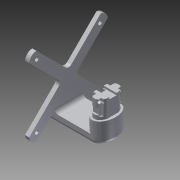
# Autodesk Inventor part: monitor-mount
Saved by Autodesk Inventor 2015 (Build 190159000, 159)
## iProperties
Created: 2015-03-06
Part Number: monitor-mount
Material: ABS Plastic
Document SubType Name: Modeling
Designer: Jody
Density: 1.06 g/cm^3
Appearance: Smooth - White
Mass: 59.874 g
Surface Area: 171.606 cm^2
Volume: 56.4849 cm^3
Author: Jody
Autodesk Inventor part; units mm, degrees
ref_plane "YZ Plane" through (0, 0, 0) normal (1, 0, 0) x (0, 1, 0)
ref_plane "XZ Plane" through (0, 0, 0) normal (0, 1, 0) x (-1, 0, 0)
ref_plane "XY Plane" through (0, 0, 0) normal (0, 0, 1) x (1, 0, 0)
sketch "Sketch1" plane through (0, 0, 0) normal (0, 1, 0) x (-1, 0, 0)
  ellipse E0 centre (0, 0) end of major axis (0, -16.9) minor radius 10.95
  dimension "d0" = 16.9
  dimension "d1" = 10.95
  constraints: 1 coincident, 2 other
extrude "Extrusion1" add sketch "Sketch1" along normal blind 25
sketch "Sketch2" plane through (0, 25, 0) normal (0, 1, 0) x (1, 0, 0)
  line L0 (7.6, 6.869) -> (7.6, -6.8693)
  line L1 (-7.6, -6.8693) -> (-7.6, 6.869)
  line L2 (1.547, -14.35) -> (-1.547, -14.35)
  line L3 (-1.547, 14.35) -> (1.547, 14.35)
  spline S0 degree 5 poles (7.6, 6.869) (7.3339, 7.69) (6.6747, 9.389) (5.6155, 11.3113) (4.2798, 12.863) (2.8086, 13.8602) (1.8557, 14.2496) (1.547, 14.35) knots 0 0 0 0 0 0 0.371815 0.797909 1 1 1 1 1 1
  line L4 (7.9552, 5.7734) -> (7.2448, 7.9647) construction
  arc A0 (7.863, 5.9868) -> (7.2954, 7.7378) centre (-10.8296, 0.8944) ccw construction
  spline S1 degree 5 poles (-1.547, 14.35) (-1.8557, 14.2496) (-2.8086, 13.8602) (-4.2798, 12.863) (-5.6155, 11.3113) (-6.6747, 9.389) (-7.3339, 7.69) (-7.6, 6.869) knots 0 0 0 0 0 0 0.202091 0.628185 1 1 1 1 1 1
  line L5 (-7.2448, 7.9647) -> (-7.9552, 5.7734) construction
  arc A1 (-7.2954, 7.7378) -> (-7.863, 5.9868) centre (10.8296, 0.8944) ccw construction
  spline S2 degree 5 poles (-7.6, -6.8693) (-7.3341, -7.6901) (-6.733, -9.2397) (-5.6943, -11.1801) (-4.3754, -12.7614) (-2.913, -13.7987) (-1.9626, -14.2149) (-1.547, -14.35) knots 0 0 0 0 0 0 0.37178 0.727887 1 1 1 1 1 1
  spline S3 degree 5 poles (1.547, -14.35) (1.9626, -14.2149) (2.913, -13.7987) (4.3754, -12.7614) (5.6943, -11.1801) (6.733, -9.2397) (7.3341, -7.6901) (7.6, -6.8693) knots 0 0 0 0 0 0 0.272113 0.62822 1 1 1 1 1 1
  line L6 (-2.5566, -14.0218) -> (-0.5374, -14.6782) construction
  arc A2 (-2.3246, -14.0283) -> (-0.7288, -14.5471) centre (0.1247, -9.2081) ccw construction
  line L7 (0.5374, -14.6782) -> (2.5566, -14.0218) construction
  arc A3 (0.7288, -14.5471) -> (2.3246, -14.0283) centre (-0.1247, -9.2081) ccw construction
  point P0 (5.4887, -11.1759)
  point P1 (2.672, 13.8453)
  point P2 (-5.4887, 11.1759)
  point P3 (-2.672, -13.8453)
  constraints: 24 end point, 8 midpoint, 4 centre point, 4 point on circle, 2 parallel, 1 horizontal, 1 perpendicular, 24 other
extrude "Extrusion3" add sketch "Sketch2" along normal blind 21
sketch "Sketch6" plane through (0, 46, 0) normal (0, 1, 0) x (1, 0, 0)
  line L0 (3.7, -9.8) -> (10.95, -9.8)
  line L1 (-10.95, -8.35) -> (-3.7, -8.35)
  line L2 (-3.7, -8.35) -> (-3.7, -16.9)
  line L3 (3.7, -9.8) -> (3.7, -16.9)
  line L4 (-3.7, -16.9) -> (-10.95, -8.35)
  line L5 (3.7, -16.9) -> (10.95, -9.8)
  line L6 (3.7, 9.8) -> (10.95, 9.8)
  line L7 (-10.95, 8.35) -> (-3.7, 8.35)
  line L8 (-3.7, 8.35) -> (-3.7, 16.9)
  line L9 (3.7, 9.8) -> (3.7, 16.9)
  line L10 (-3.7, 16.9) -> (-10.95, 8.35)
  line L11 (3.7, 16.9) -> (10.95, 9.8)
  point P0 (0, 0)
  constraints: 24 end point
extrude "Extrusion4" cut sketch "Sketch6" against normal blind 17.7
sketch "Sketch7" plane through (0, 46, 0) normal (0, 1, 0) x (1, 0, 0)
  ellipse E0 centre (0, 0) end of major axis (0, -16.9) minor radius 10.95 projected
  line L0 (10.581, -4.35) -> (-10.581, -4.35)
  line L1 (-10.581, -4.35) -> (-10.581, 4.35)
  line L2 (-10.581, 4.35) -> (10.581, 4.35)
  line L3 (10.581, 4.35) -> (10.581, -4.35)
  line L4 (10.581, -4.35) -> (-10.581, 4.35) construction
  line L5 (-10.581, -4.35) -> (10.581, 4.35) construction
  dimension "d23" = 8.7
  constraints: 12 end point, 2 midpoint, 2 parallel, 1 horizontal, 1 perpendicular, 2 other
  measures "d23" distance of L0.end L1.end
extrude "Extrusion5" cut sketch "Sketch7" against normal blind 2.4 contours L0 L1 L2 L3
sketch "Sketch8" plane through (7.6, 25, 6.8693) normal (1, 0, 0) x (0, 0, -1)
  line L0 (-7.4807, 4.8) -> (-7.4807, 12.1)
  line L1 (-5.4807, 4.8) -> (-5.4807, 12.1)
  line L2 (-7.4807, 4.8) -> (-5.4807, 4.8)
  line L3 (-5.4807, 12.1) -> (-7.4807, 12.1)
  line L4 (21.2193, 4.8) -> (21.2193, 12.1)
  line L5 (19.2193, 4.8) -> (19.2193, 12.1)
  line L6 (21.2193, 4.8) -> (19.2193, 4.8)
  line L7 (19.2193, 12.1) -> (21.2193, 12.1)
  point P0 (6.8693, -25)
  point P1 (0, 0)
  constraints: 16 end point, 2 horizontal
extrude "Extrusion6" cut sketch "Sketch8" against normal up to next
sketch "Sketch9" plane through (-7.6, 25, -6.869) normal (-1, 0, 0) x (0, 0, 1)
  line L0 (3.4692, 5) -> (10.2692, 5)
  line L1 (3.4692, 5) -> (3.4692, 18.6)
  line L2 (10.2692, 5) -> (10.2692, 18.6)
  line L3 (3.4692, 18.6) -> (10.2692, 18.6)
  point P0 (6.869, -25)
  constraints: 8 end point, 1 perpendicular
extrude "Extrusion7" cut sketch "Sketch9" against normal blind 3.5
sketch "Sketch10" plane through (-7.6, 30, -3.3999) normal (0, 0, 1) x (1, 0, 0)
  line L0 (0, 0) -> (3.5, 7.1937)
  line L1 (3.5, 0) -> (3.5, 13.6) projected
  line L2 (3.5, 7.1937) -> (3.5, 8.6937)
  line L3 (3.5, 8.6937) -> (0.864, 10.4946)
  line L4 (0, 0) -> (3.5, 0)
  line L5 (0, 0) -> (3.5, 0) projected
  line L6 (0.864, 10.4946) -> (3.5, 13.6)
  point P0 (7.6, -30)
  dimension "d36" = 8
  dimension "d37" = 1.5
  constraints: 10 end point, 2 point on line, 1 collinear
  measures "d36" distance of L0.start L0.end
  measures "d37" distance of L0.end L2.end
extrude "Extrusion8" add sketch "Sketch10" along normal up to next
fillet "Fillet1" radius 0.5 1 edges at (-6.736, 40.4946, 0.0001)
sketch "Sketch11" plane through (3.7, 46, 13.1272) normal (1, 0, 0) x (0, 0, -1)
  circle A0 centre (1.6989, -3.0978) radius 2.25
  line L0 (17.4772, -2.4) -> (8.7772, -2.4) projected
  line L1 (16.5271, -2.4) -> (9.7271, -2.4) projected
  circle A1 centre (24.5552, -3.0978) radius 2.25
  point P0 (13.1272, -46)
  dimension "d43" = 4.5
  constraints: 2 centre point
  measures "d43" diameter of A0
extrude "Extrusion9" cut sketch "Sketch11" along normal blind 10 and the other way blind 5
sketch "Sketch12" plane through (0, 0, 0) normal (0, -1, 0) x (1, 0, 0)
  ellipse E0 centre (0, 0) end of major axis (0, 16.9) minor radius 10.95 projected
  line L0 (0, 16.9) -> (0, -16.9)
  line L1 (0, -16.9) -> (-50, -16.9)
  line L2 (-50, -16.9) -> (-50, 16.9)
  line L3 (-50, 16.9) -> (0, 16.9)
  dimension "d50" = 50
  constraints: 8 end point, 2 parallel, 1 perpendicular, 1 vertical, 3 other
  measures "d50" distance of L0.end L1.end
extrude "Extrusion10" add sketch "Sketch12" against normal blind 10 contours E0 L1 L2 L3
sketch "Sketch13" plane through (-50, 0, -16.9) normal (-1, 0, 0) x (0, 0, 1)
  circle A0 centre (54.4, 75.1899) radius 2.25
  line L0 (25.3853, 37.6899) -> (63.569, 75.8737)
  line L1 (16.9, 46.1752) -> (55.0838, 84.359)
  arc A1 (63.569, 75.8737) -> (55.0838, 84.359) centre (54.4, 75.1899) ccw
  circle A2 centre (-20.6, 75.1899) radius 2.25
  line L2 (16.9, 46.1752) -> (-21.2838, 84.359)
  line L3 (8.4147, 37.6899) -> (-29.769, 75.8737)
  arc A3 (-21.2838, 84.359) -> (-29.769, 75.8737) centre (-20.6, 75.1899) ccw
  circle A4 centre (54.4, 75.1899) radius 2.25
  line L4 (8.4147, 37.6899) -> (-29.769, -0.4938)
  line L5 (16.9, 29.2046) -> (-21.2838, -8.9791)
  arc A5 (-29.769, -0.4938) -> (-21.2838, -8.9791) centre (-20.6, 0.1899) ccw
  circle A6 centre (54.4, 0.1899) radius 2.25
  line L6 (16.9, 29.2046) -> (55.0838, -8.9791)
  line L7 (25.3853, 37.6899) -> (63.569, -0.4938)
  arc A7 (55.0838, -8.9791) -> (63.569, -0.4938) centre (54.4, 0.1899) ccw
  circle A8 centre (-20.6, 0.1899) radius 2.25
  point P0 (16.9, 37.6899)
  point P1 (16.9, 37.6899)
  point P2 (16.9, 37.6899)
  point P3 (16.9, 37.6899)
  dimension "d58" = 4.5
  dimension "d63" = 4.5
  dimension "d64" = 4.5
  dimension "d65" = 4.5
  dimension "d66" = 4.5
  dimension "d67" = 75
  dimension "d68" = 75
  constraints: 16 end point, 9 centre point, 8 point on circle, 3 coincident
  measures "d58" diameter of A0
  measures "d63" diameter of A2
  measures "d64" diameter of A4
  measures "d65" diameter of A6
  measures "d66" diameter of A8
  measures "d67" distance of A0.centre A2.centre
  measures "d68" distance of A6.centre A1.centre
extrude "Extrusion11" add sketch "Sketch13" against normal blind 5
fillet "Fillet2" radius 5 4 edges at (-47.5, 46.1752, 0) (-47.5, 29.2046, 0) (-47.5, 37.6899, -8.4853) (-47.5, 37.6899, 8.4853)
sketch "Sketch14" plane through (0, 10, 0) normal (0, 1, 0) x (1, 0, 0)
  line L0 (-45, -16.9) -> (-50, -16.9)
  line L1 (-45, 16.9) -> (-45, -16.9)
  line L2 (-45, 16.9) -> (-50, 16.9)
  line L3 (-50, 16.9) -> (-50, -16.9)
  point P0 (0, 0)
  point P1 (-50, 14.2046)
  constraints: 8 end point, 2 horizontal, 2 point on line, 1 perpendicular
extrude "Extrusion12" add sketch "Sketch14" along normal up to next
fillet "Fillet4" radius 5 3 edges at (10.95, 0, 0) (-25, 0, 16.9) (-25, 0, -16.9)
fillet "Fillet5" radius 5 1 edges at (-45, 10, 0)
sketch "Sketch15" plane through (0, 10, 0) normal (0, 1, 0) x (1, 0, 0)
  point P0 (0, 0)
body "Solid1"
